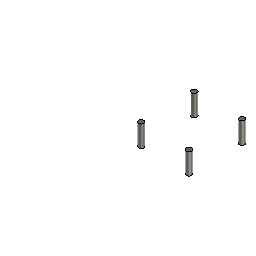
Pin (Autodesk Fusion 360 design; units mm, degrees)
Autodesk Fusion 360 part; units mm, degrees
sketch "Sketch1" plane through (0, 0, 50) normal (0, 0, 1) x (-1, 0, 0)
  circle A0 centre (-55, 5) radius 2.5
  circle A1 centre (-55, -45) radius 2.5
  circle A2 centre (-10, 5) radius 2.5
  circle A3 centre (-10, -45) radius 2.5
  line L0 (10, 10) -> (-75, 10)
  line L1 (-75, 10) -> (-75, -50)
  line L2 (-75, -50) -> (10, -50)
  line L3 (10, -50) -> (10, 10)
  circle A4 centre (-10, -45) radius 2.5
  circle A5 centre (-55, -45) radius 2.5
  circle A6 centre (-55, 5) radius 2.5
  circle A7 centre (-10, 5) radius 2.5
  constraint concentric A3 A4
  constraint concentric A1 A5
  constraint concentric A0 A6
  constraint concentric A2 A7
extrude "Extrude1" add sketch "Sketch1" against normal blind 20 contours A0 A6 | A1 A5 | A2 A7 | A3 A4 makes body 1 at (52.5031, -4.8754, 36.6667) makes body 2 at (52.5031, 45.1246, 36.6667) makes body 3 at (7.5031, -4.8754, 36.6667) makes body 4 at (7.5031, 45.1246, 36.6667)
